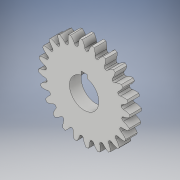
# Autodesk Inventor part: SpurGear
Saved by Autodesk Inventor 2019.3 (Build 233278000, 278)
## iProperties
Created: 2019-09-04
Part Number: SpurGear
Material: Generic
Document SubType Name: Modeling
Designer: Frienddo
Density: 1 g/cm^3
Appearance: Default
Author: Frienddo
Autodesk Inventor part; units mm, degrees
ref_plane "YZ Plane" through (0, 0, 0) normal (1, 0, 0) x (0, 1, 0)
ref_plane "XZ Plane" through (0, 0, 0) normal (0, 1, 0) x (-1, 0, 0)
ref_plane "XY Plane" through (0, 0, 0) normal (0, 0, 1) x (1, 0, 0)
sketch "Base" plane through (0, 0, 0) normal (0, 0, 1) x (1, 0, 0)
  circle A0 centre (0, 0) radius 32.25 construction
  circle A1 centre (0, 0) radius 33.8289 construction
  circle A2 centre (0, 0) radius 36 construction
  circle A3 centre (0, 0) radius 39 construction
  line L0 (31.7888, 11.5702) -> (36, 0) construction
  line L1 (-56.1201, 0) -> (63.7209, 0) construction
  line L2 (31.7888, 11.5702) -> (0, 0) construction
  line L3 (36, 0) -> (46.6007, 3.8583) construction
  arc A4 (33.8238, -0.5872) -> (38.9699, 1.5311) centre (31.4865, 12.4008) ccw
  line L4 (38.9699, 1.5311) -> (38.8364, 3.5686)
  arc A5 (38.8364, 3.5686) -> (33.4578, 4.9971) centre (32.8357, -8.1849) ccw
  line L5 (33.4578, 4.9971) -> (31.8962, 4.7639)
  line L6 (31.2913, 7.8049) -> (0, 0)
  line L7 (33.8238, -0.5872) -> (0, 0)
  line L8 (35.692, 4.6989) -> (0, 0) construction
  line L9 (38.9032, 2.5498) -> (0, 0) construction
  line L10 (38.8364, 3.5686) -> (0, 0) construction
  line L11 (38.9699, 1.5311) -> (0, 0) construction
  arc A6 (32.8233, 8.187) -> (31.6283, 6.302) centre (33.2148, 6.6176) ccw
  line L12 (33.2148, 6.6176) -> (32.8233, 8.187) construction
  line L13 (33.2148, 6.6176) -> (31.6283, 6.302) construction
  line L14 (32.8233, 8.187) -> (31.2913, 7.8049)
  arc A7 (31.6324, 6.2814) -> (33.4578, 4.9971) centre (33.2189, 6.5969) ccw
  line L15 (33.2189, 6.5969) -> (33.4578, 4.9971) construction
  line L16 (33.2189, 6.5969) -> (31.6324, 6.2814) construction
  line L17 (31.6324, 6.2814) -> (31.6283, 6.302)
  line L18 (31.6303, 6.2917) -> (0, 0) construction
  circle A8 centre (0, 0) radius 12.5
  line L19 (0, -54.6) -> (0, 54.6) construction
  line L20 (2.5, 9.2474) -> (-2.5, 9.2474)
  line L21 (-2.5, 9.2474) -> (-2.5, 15.2474)
  line L22 (-2.5, 15.2474) -> (2.5, 15.2474)
  line L23 (2.5, 15.2474) -> (2.5, 9.2474)
  line L24 (2.5, 9.2474) -> (-2.5, 15.2474) construction
  line L25 (-2.5, 9.2474) -> (2.5, 15.2474) construction
  line L26 (-2.5, 12.2474) -> (2.5, 12.2474) construction
  point P0 (0, 12.2474)
  dimension "sdTemp" = 25
  dimension "RefDiam" = 72
  dimension "RootDiam" = 64.5
  dimension "BaseDiam" = 67.6579
  dimension "TipDiam" = 78
  dimension "Pitch" = 15
  dimension "ToothThick" = 7.5
  dimension "InnerToothThick" = 3
  dimension "kwdTemp" = 3
  dimension "kwTemp" = 5
  dimension "khTemp" = 6
  constraints: 50 end point, 21 point on circle, 8 centre point, 6 coincident, 6 midpoint, 6 tangent, 4 perpendicular, 2 parallel, 2 point on line, 1 collinear, 1 horizontal, 6 other
  measures "RefDiam" diameter of A2
  measures "RootDiam" diameter of A0
  measures "BaseDiam" diameter of A1
  measures "TipDiam" diameter of A3
  measures "Pitch" angle of L7 L6
  measures "ToothThick" angle of L1 L8
  measures "InnerToothThick" angle of L11 L10
  measures "kwdTemp" distance between parallel lines of L22 L26
  measures "kwTemp" distance of L21.end L22.end
  measures "khTemp" distance of L20.end L21.end
extrude "GearOneTooth" add sketch "Base" along normal mid plane 10 contours L7 A8 L6 L14 A6 L17 A7 A5 L4 A4 | L7 L6 A8
pattern_circular "GearCircularPattern" count 24 over 360 about axis through (0, 0, -10) along (0, 0, 1) of "GearOneTooth"
extrude "Shaft" cut sketch "Base" along normal mid plane 10 contours A8 L21 L20 L23 L6 L7 | L7 L6 A8 | L21 L22 L23 A8 | A8 L23 L20 L21
equation "\"RootDiam\" = RefDiam - 2.5 * Module"
equation "\"TipDiam\" = RefDiam + 2 * Module"
equation "\"ToothThick\" = 0.5 * Pitch"
equation "\"InnerToothThick\" = 0.2 * Pitch"
equation "\"Module\" = 3"
equation "\"ReferencePressureAngle\" = 20deg"
equation "\"ShaftDiameter\" = 25"
equation "\"KeyWidth\" = 5"
equation "\"KeyHeight\" = 6"
equation "\"KeywayDepth\" = 3"
body "Solid1"
